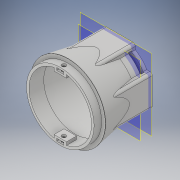
# Autodesk Inventor part: endkappen_V4
Saved by Autodesk Inventor 2017 (Build 210142000, 142)
## iProperties
Part Number: endkappen_V4
Material: Generisch
Document SubType Name: Modeling
Designer: Fabio
Density: 1 g/cm^3
Appearance: Vorgabe
Author: Fabio
Autodesk Inventor part; units mm, degrees
ref_plane "YZ Plane" through (0, 0, 0) normal (1, 0, 0) x (0, 1, 0)
ref_plane "XZ Plane" through (0, 0, 0) normal (0, 1, 0) x (-1, 0, 0)
ref_plane "XY Plane" through (0, 0, 0) normal (0, 0, 1) x (1, 0, 0)
sketch "Skizze2" plane through (0, 0, 0) normal (1, 0, 0) x (0, 1, 0)
  line L0 (0, 0) -> (48.6481, 0)
  line L1 (47.4748, 20) -> (47.4748, 25)
  line L2 (6, 30) -> (6, 27)
  line L3 (6, 27) -> (0, 27)
  line L4 (6.2626, 30) -> (6, 30)
  line L5 (11.7576, 25) -> (0, 25)
  line L6 (0, 25) -> (0, 27)
  line L7 (0, 0) -> (0, 25) construction
  line L8 (40.5337, 20) -> (47.4748, 20)
  line L9 (11.7576, 25) -> (40.5337, 20)
  line L10 (47.4748, 25) -> (35.0388, 25)
  line L11 (6.2626, 30) -> (35.0388, 25)
  dimension "d164" = 60
  dimension "d166" = 54
  dimension "d167" = 50
  dimension "d168" = 6
  dimension "d171" = 47.4748
  dimension "d174" = 40.5337
  dimension "d203" = 3
  dimension "d204" = 40
  dimension "d205" = 5
  dimension "d206" = 170.143
  dimension "d207" = 12.436
  constraints: 24 end point, 5 horizontal, 2 vertical, 1 parallel, 1 perpendicular
  measures "d164" diameter of L4 L0
  measures "d166" diameter of L3 L0
  measures "d167" diameter of L5 L0
  measures "d168" distance of L2.end L3.end
  measures "d171" distance of L5.end L1.end
  measures "d174" distance from line of L7 L8.start
  measures "d203" distance of L2.start L2.end
  measures "d204" diameter of L8 L0
  measures "d205" distance of L1.start L1.end
  measures "d206" angle of L5 L9
  measures "d207" distance of L1.end L10.end
revolve "Umdrehung1" add sketch "Skizze2" angle 360 about axis through (0, 0, 0) along (0, 1, 0)
sketch "Skizze18" plane through (0, 0, 0) normal (0, -1, 0) x (1, 0, 0)
  circle A0 centre (0, 0) radius 25 projected
  line L0 (5, -22) -> (-5, -22)
  line L1 (-5, -22) -> (-5, -25)
  line L2 (-5, -25) -> (5, -25)
  line L3 (5, -25) -> (5, -22)
  line L4 (5, -22) -> (-5, -25) construction
  line L5 (-5, -22) -> (5, -25) construction
  line L6 (0, -23.5) -> (0, 0) construction
  line L7 (0, 0) -> (9.0804, 0) construction
  line L8 (5, 22) -> (-5, 22)
  line L9 (-5, 22) -> (-5, 25)
  line L10 (-5, 25) -> (5, 25)
  line L11 (5, 25) -> (5, 22)
  dimension "d176" = 10
  dimension "d177" = 3
  dimension "d178" = 22
  constraints: 24 end point, 4 symmetric about line, 2 horizontal, 2 midpoint, 2 parallel, 1 perpendicular, 1 vertical
  measures "d176" distance of L2.end L1.end
  measures "d177" distance of L0.end L1.end
  measures "d178" distance from line of point (0, 0) L0
extrude "Extrusion14" add sketch "Skizze18" against normal blind 8 contours L11 L8 L9 A0 | A0 L10 L11 | L3 L2 A0 | A0 L1 L0 L3 | A0 L9 L10 | L2 L1 A0
sketch "Skizze19" plane through (0, 0, 0) normal (0, -1, 0) x (1, 0, 0)
  arc A0 (-5, -24.4949) -> (5, -24.4949) centre (0, 0) ccw projected
  line L0 (0, 0) -> (9.7237, 0) construction
  line L1 (0, -24.5) -> (0, 0) construction
  line L2 (2.85, -23.5) -> (-2.85, -23.5)
  line L3 (-2.85, -23.5) -> (-2.85, -25.5)
  line L4 (-2.85, -25.5) -> (2.85, -25.5)
  line L5 (2.85, -25.5) -> (2.85, -23.5)
  line L6 (2.85, -23.5) -> (-2.85, -25.5) construction
  line L7 (-2.85, -23.5) -> (2.85, -25.5) construction
  line L8 (2.85, 23.5) -> (-2.85, 23.5)
  line L9 (-2.85, 23.5) -> (-2.85, 25.5)
  line L10 (-2.85, 25.5) -> (2.85, 25.5)
  line L11 (2.85, 25.5) -> (2.85, 23.5)
  dimension "d236" = 5.7
  dimension "d237" = 2
  dimension "d238" = 23.5
  constraints: 24 end point, 4 symmetric about line, 2 horizontal, 2 midpoint, 2 parallel, 1 perpendicular, 1 vertical
  measures "d236" distance of L4.end L3.end
  measures "d237" distance of L3.end L2.end
  measures "d238" distance between parallel lines of L0 L2
extrude "Extrusion15" cut sketch "Skizze19" against normal blind 5.7
sketch "Skizze20" plane through (5, 0, 22) normal (0, 0, -1) x (-1, 0, 0)
  line L0 (10, 0) -> (0, 0) projected
  line L1 (10, 0) -> (10, 8) projected
  point P0 (5, 0)
  point P1 (5, 2.85)
  dimension "d185" = 2.85
  dimension "d186" = 5
  measures "d185" distance from line of L0 point (5, 2.85)
  measures "d186" distance from line of L1 point (5, 2.85)
hole "Bohrung4" at (0, 2.85, 22) direction (0, 0, 1) diameter 3.3 end through all
sketch "Skizze21" plane through (-5, 0, -22) normal (0, 0, 1) x (1, 0, 0)
  line L0 (10, 0) -> (0, 0) projected
  line L1 (0, 0) -> (0, 8) projected
  point P0 (5, 0)
  point P1 (5, 2.85)
  dimension "d194" = 2.85
  dimension "d195" = 5
  measures "d194" distance from line of point (5, 2.85) L0
  measures "d195" distance from line of L1 point (5, 2.85)
hole "Bohrung5" at (0, 2.85, -22) direction (0, 0, -1) diameter 3.3 end through all
sketch "Skizze25" plane through (0, 47.4748, 0) normal (0, 1, 0) x (1, 0, 0)
  circle A0 centre (0, 0) radius 25 projected
  line L0 (22.5, 22.5) -> (-22.5, 22.5) construction
  line L1 (-22.5, 22.5) -> (-22.5, -22.5) construction
  line L2 (-22.5, -22.5) -> (22.5, -22.5) construction
  line L3 (22.5, -22.5) -> (22.5, 22.5) construction
  line L4 (22.5, 22.5) -> (-22.5, -22.5) construction
  line L5 (-22.5, 22.5) -> (22.5, -22.5) construction
  line L6 (12.5, -21.5) -> (-12.5, -21.5)
  line L7 (-12.5, -21.5) -> (-12.5, -26)
  line L8 (-12.5, -26) -> (12.5, -26)
  line L9 (12.5, -26) -> (12.5, -21.5)
  line L10 (12.5, -21.5) -> (-12.5, -26) construction
  line L11 (-12.5, -21.5) -> (12.5, -26) construction
  line L12 (26, -12.5) -> (26, 12.5)
  line L13 (21.5, -12.5) -> (26, -12.5)
  line L14 (21.5, 12.5) -> (21.5, -12.5)
  line L15 (26, 12.5) -> (21.5, 12.5)
  line L16 (12.5, 26) -> (-12.5, 26)
  line L17 (12.5, 21.5) -> (12.5, 26)
  line L18 (-12.5, 21.5) -> (12.5, 21.5)
  line L19 (-12.5, 26) -> (-12.5, 21.5)
  line L20 (-26, 12.5) -> (-26, -12.5)
  line L21 (-21.5, 12.5) -> (-26, 12.5)
  line L22 (-21.5, -12.5) -> (-21.5, 12.5)
  line L23 (-26, -12.5) -> (-21.5, -12.5)
  point P0 (0, -23.75)
  dimension "d243" = 45
  dimension "d244" = 45
  dimension "d246" = 4.5
  dimension "d247" = 25
  dimension "d248" = 21.5
  dimension "d251" = 360
  dimension "d255" = 23.75
  constraints: 48 end point, 4 midpoint, 4 parallel, 2 horizontal, 2 perpendicular, 33 other
  measures "d243" distance of L2.end L1.end
  measures "d244" distance of L1.end L0.end
  measures "d246" distance of L6.end L7.end
  measures "d247" distance of L7.end L8.end
  measures "d248" distance from line of point (0, 0) L6
  measures "d255" distance of point (0, 0) point (0, -23.75)
extrude "Extrusion18" add sketch "Skizze25" against normal blind 35 contours A0 L13 L14 L15 | A0 L15 L12 L13 | L17 L18 L19 A0 | A0 L19 L16 L17 | L9 L8 L7 A0 | A0 L7 L6 L9 | L21 L22 L23 A0 | A0 L23 L20 L21
delete faces "Fläche löschen11" heal yes whole lump no faces at (-22.2148, 12.4748, -2.576) (-21.5, 18.3986, -3.4181)
delete faces "Fläche löschen12" heal yes whole lump no faces at (22.2148, 12.4748, 2.576) (21.5, 18.3986, 3.4181)
delete faces "Fläche löschen13" heal yes whole lump no faces at (-2.851, 12.4748, 22.1196) (-2.848, 15.8345, 21.5)
delete faces "Fläche löschen14" heal yes whole lump no faces at (0.8715, 12.4748, -22.5792) (3.4181, 18.3986, -21.5)
ref_plane "Arbeitsebene4" through (-12.5, 44.4748, -26) normal (0, 1, 0) x (1, 0, 0)
sketch "Skizze26" plane through (-12.5, 44.4748, -26) normal (0, 1, 0) x (1, 0, 0)
  line L0 (-10, -48.5) -> (35, -48.5)
  line L1 (35, -48.5) -> (35, -3.5)
  line L2 (35, -3.5) -> (-10, -3.5)
  line L3 (-10, -3.5) -> (-10, -48.5)
  line L4 (-10, -48.5) -> (35, -3.5) construction
  line L5 (35, -48.5) -> (-10, -3.5) construction
  line L6 (-10, -3.5) -> (-10, 8.0726)
  line L7 (-10, 8.0726) -> (35, 8.0726)
  line L8 (35, 8.0726) -> (35, -3.5)
  point P0 (12.5, -26)
  dimension "d257" = 45
  dimension "d258" = 45
  dimension "d259" = 11.5726
  constraints: 18 end point, 3 perpendicular, 2 midpoint, 2 parallel, 1 horizontal, 1 vertical
  measures "d257" distance of L2.end L1.end
  measures "d258" distance of L1.end L0.end
  measures "d259" distance between parallel lines of L7 L2
fillet "Rundung2" radius 2 8 edges at (26, 30.1816, -12.5) (26, 30.1816, 12.5) (12.5, 30.1816, 26) (-26, 30.1816, -12.5) (-12.5, 30.1816, -26) (12.5, 30.1816, -26) (-12.5, 30.1816, 26) (-26, 30.1816, 12.5)
sketch "Skizze29" plane through (-10.5, 47.4748, 26) normal (0, 1, 0) x (1, 0, 0)
  line L0 (0, 52) -> (21, 52) projected
  circle A0 centre (10.5, 52) radius 2.5
  point P0 (10.5, 26)
  dimension "d276" = 5
  constraints: 1 centre point, 1 midpoint
  measures "d276" diameter of A0
extrude "Extrusion22" add sketch "Skizze29" against normal blind 34
delete faces "Fläche löschen15" heal yes whole lump no faces at (-0.3409, 15.7084, -23.5233) (0, 13.4748, -24.2946)
extrude "Extrusion23" cut sketch "Skizze26" against normal blind 2.5
sketch "Skizze30" plane through (-10.5, 47.4748, 26) normal (0, 1, 0) x (1, 0, 0)
  arc A0 (13, 52) -> (8, 52) centre (10.5, 52) ccw projected
  point P0 (10.5, 26)
  constraints: 1 coincident
hole "Bohrung8" at (0, 47.4748, -26) direction (0, -1, 0) diameter 3.3 depth 15 tip angle 118
ref_plane "Arbeitsebene5" through (-12.5, 38.9748, -26) normal (0, 1, 0) x (1, 0, 0)
sketch "Skizze31" plane through (-12.5, 38.9748, -26) normal (0, 1, 0) x (1, 0, 0)
  circle A0 centre (12.5, 0) radius 1.65 projected
  line L0 (15.35, 2.85) -> (9.65, 2.85)
  line L1 (9.65, 2.85) -> (9.65, -2.85)
  line L2 (9.65, -2.85) -> (15.35, -2.85)
  line L3 (15.35, -2.85) -> (15.35, 2.85)
  line L4 (15.35, 2.85) -> (9.65, -2.85) construction
  line L5 (9.65, 2.85) -> (15.35, -2.85) construction
  point P0 (12.5, -26)
  dimension "d289" = 5.7
  dimension "d290" = 5.7
  constraints: 12 end point, 2 midpoint, 2 parallel, 1 horizontal, 1 perpendicular
  measures "d289" distance of L2.end L1.end
  measures "d290" distance of L1.end L0.end
extrude "Extrusion24" cut sketch "Skizze31" against normal blind 2
